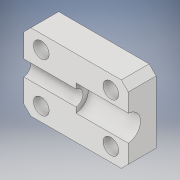
# Autodesk Inventor part: Piston driver clamp
Saved by Autodesk Inventor 2018 (Build 220112000, 112)
## iProperties
Created: 2013-11-24
Part Number: Piston driver clamp
Material: ASA Plastic
Document SubType Name: Modeling
Designer: Gabriel Smolnycki
Mass: 4.60248 g
Surface Area: 24.984 cm^2
Volume: 4.30138 cm^3
Density: 1.07 g/cm^3
Appearance: Smooth - White ASA
Sending System: SolidWorks 2017
Last Author: Gabriel Smolnycki
Last Saved: 2017-09-14
Author: Gabriel Smolnycki
Autodesk Inventor part; units mm, degrees
ref_plane "XZ Plane" through (0, 0, 0) normal (0, 1, 0) x (-1, 0, 0)
ref_plane "XY Plane" through (0, 0, 0) normal (0, 0, 1) x (1, 0, 0)
ref_plane "Work Plane1" through (-15, 0, 0) normal (1, 0, 0) x (0, 1, 0)
sketch "Sketch1" plane through (-15, 0, 0) normal (1, 0, 0) x (0, 1, 0)
  line L0 (11, 0) -> (-11, 0)
  line L1 (11, 8) -> (11, 0)
  line L2 (11, 8) -> (2.2361, 8)
  line L3 (-11, 8) -> (-11, 0)
  line L4 (-2.2361, 8) -> (-11, 8)
  arc A0 (-2.2361, 8) -> (2.2361, 8) centre (0, 8.25) ccw
  constraints: 10 end point, 3 horizontal, 2 equal length, 2 point on circle, 2 vertical, 1 centre point
extrude "Extrusion2" add sketch "Sketch1" along normal blind 30
sketch "Sketch2" plane through (15, 0, 0) normal (1, 0, 0) x (0, 0, -1)
  line L0 (-8, -2.2361) -> (-8, -3.7417)
  arc A0 (-8, -2.2361) -> (-8, 2.2361) centre (-8.25, 0) ccw
  arc A1 (-8, -3.7417) -> (-8, 3.7417) centre (-8.25, 0) ccw
  line L1 (-8, 3.7417) -> (-8, 2.2361)
  constraints: 4 end point, 4 point on circle, 2 centre point, 2 collinear, 2 vertical
extrude "Extrusion1" cut sketch "Sketch2" against normal blind 15
hole "Hole4" at (10, -7, 8) direction (0, 0, -1) diameter 4.5 depth 8
hole "Hole3" at (10, 7, 8) direction (0, 0, -1) diameter 4.5 depth 8
sketch "Sketch4" plane through (-15, -11, 8) normal (0, 0, 1) x (1, 0, 0)
  point P0 (25, 18)
hole "Hole2" at (-10, -7, 8) direction (0, 0, -1) diameter 4.5 depth 8
sketch "Sketch3" plane through (-15, -11, 8) normal (0, 0, 1) x (1, 0, 0)
  point P0 (25, 4)
hole "Hole1" at (-10, 7, 8) direction (0, 0, -1) diameter 4.5 depth 8
chamfer "Chamfer4" distance 2 angle 45 1 edges at (-15, -11, 4)
chamfer "Chamfer3" distance 2 angle 45 1 edges at (15, -11, 4)
chamfer "Chamfer2" distance 2 angle 45 1 edges at (-15, 11, 4)
chamfer "Chamfer1" distance 2 angle 45 1 edges at (15, 11, 4)
sketch "Sketch5" plane through (-15, -11, 8) normal (0, 0, 1) x (1, 0, 0)
  point P0 (5, 4)
sketch "Sketch6" plane through (-15, -11, 8) normal (0, 0, 1) x (1, 0, 0)
  point P0 (5, 18)
body "Solid3"
